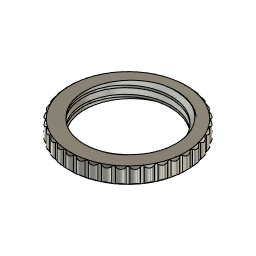
M12x1 knurled thumb nut (Autodesk Fusion 360 design; units mm, degrees)
Autodesk Fusion 360 part; units mm, degrees
sketch "Sketch1" plane through (0, 0, 0) normal (0, 0, 1) x (1, 0, 0)
  circle A0 centre (0, 0) radius 6
  circle A1 centre (0, 0) radius 7.35 construction
  circle A2 centre (0, 0) radius 7.5 construction
  line L0 (0, 0) -> (0, 8.1) construction
  arc A3 (-0.8115, 7.3051) -> (-0.4693, 7.335) centre (-0.6628, 7.5762) ccw
  arc A4 (0, 7.5) -> (-0.4693, 7.335) centre (0, 6.75) ccw
  arc A5 (-0.8115, 7.3051) -> (-1.3024, 7.3861) centre (-1.1721, 6.6475) ccw
  arc A6 (-2.0677, 7.0532) -> (-2.5652, 7.0477) centre (-2.3086, 6.3429) ccw
  arc A7 (-2.0677, 7.0532) -> (-1.7359, 7.1421) centre (-1.9684, 7.346) ccw
  arc A8 (-1.3024, 7.3861) -> (-1.7359, 7.1421) centre (-1.1721, 6.6475) ccw
  arc A9 (-3.261, 6.587) -> (-3.75, 6.4952) centre (-3.375, 5.8457) ccw
  arc A10 (-3.261, 6.587) -> (-2.9497, 6.7321) centre (-3.2141, 6.8926) ccw
  arc A11 (-2.5652, 7.0477) -> (-2.9497, 6.7321) centre (-2.3086, 6.3429) ccw
  arc A12 (-4.3553, 5.9206) -> (-4.8209, 5.7453) centre (-4.3388, 5.1708) ccw
  arc A13 (-4.3553, 5.9206) -> (-4.074, 6.1176) centre (-4.3621, 6.2298) ccw
  arc A14 (-3.75, 6.4952) -> (-4.074, 6.1176) centre (-3.375, 5.8457) ccw
  arc A15 (-5.3173, 5.0744) -> (-5.7453, 4.8209) centre (-5.1708, 4.3388) ccw
  arc A16 (-5.3173, 5.0744) -> (-5.0744, 5.3173) centre (-5.3776, 5.3776) ccw
  arc A17 (-4.8209, 5.7453) -> (-5.0744, 5.3173) centre (-4.3388, 5.1708) ccw
  arc A18 (-6.1176, 4.074) -> (-6.4952, 3.75) centre (-5.8457, 3.375) ccw
  arc A19 (-6.1176, 4.074) -> (-5.9206, 4.3553) centre (-6.2298, 4.3621) ccw
  arc A20 (-5.7453, 4.8209) -> (-5.9206, 4.3553) centre (-5.1708, 4.3388) ccw
  arc A21 (-6.7321, 2.9497) -> (-7.0477, 2.5652) centre (-6.3429, 2.3086) ccw
  arc A22 (-6.7321, 2.9497) -> (-6.587, 3.261) centre (-6.8926, 3.2141) ccw
  arc A23 (-6.4952, 3.75) -> (-6.587, 3.261) centre (-5.8457, 3.375) ccw
  arc A24 (-7.1421, 1.7359) -> (-7.3861, 1.3024) centre (-6.6475, 1.1721) ccw
  arc A25 (-7.1421, 1.7359) -> (-7.0532, 2.0677) centre (-7.346, 1.9684) ccw
  arc A26 (-7.0477, 2.5652) -> (-7.0532, 2.0677) centre (-6.3429, 2.3086) ccw
  arc A27 (-7.335, 0.4693) -> (-7.5, 0) centre (-6.75, 0) ccw
  arc A28 (-7.335, 0.4693) -> (-7.3051, 0.8115) centre (-7.5762, 0.6628) ccw
  arc A29 (-7.3861, 1.3024) -> (-7.3051, 0.8115) centre (-6.6475, 1.1721) ccw
  arc A30 (-7.3051, -0.8115) -> (-7.3861, -1.3024) centre (-6.6475, -1.1721) ccw
  arc A31 (-7.3051, -0.8115) -> (-7.335, -0.4693) centre (-7.5762, -0.6628) ccw
  arc A32 (-7.5, 0) -> (-7.335, -0.4693) centre (-6.75, 0) ccw
  arc A33 (-7.0532, -2.0677) -> (-7.0477, -2.5652) centre (-6.3429, -2.3086) ccw
  arc A34 (-7.0532, -2.0677) -> (-7.1421, -1.7359) centre (-7.346, -1.9684) ccw
  arc A35 (-7.3861, -1.3024) -> (-7.1421, -1.7359) centre (-6.6475, -1.1721) ccw
  arc A36 (-6.587, -3.261) -> (-6.4952, -3.75) centre (-5.8457, -3.375) ccw
  arc A37 (-6.587, -3.261) -> (-6.7321, -2.9497) centre (-6.8926, -3.2141) ccw
  arc A38 (-7.0477, -2.5652) -> (-6.7321, -2.9497) centre (-6.3429, -2.3086) ccw
  arc A39 (-5.9206, -4.3553) -> (-5.7453, -4.8209) centre (-5.1708, -4.3388) ccw
  arc A40 (-5.9206, -4.3553) -> (-6.1176, -4.074) centre (-6.2298, -4.3621) ccw
  arc A41 (-6.4952, -3.75) -> (-6.1176, -4.074) centre (-5.8457, -3.375) ccw
  arc A42 (-5.0744, -5.3173) -> (-4.8209, -5.7453) centre (-4.3388, -5.1708) ccw
  arc A43 (-5.0744, -5.3173) -> (-5.3173, -5.0744) centre (-5.3776, -5.3776) ccw
  arc A44 (-5.7453, -4.8209) -> (-5.3173, -5.0744) centre (-5.1708, -4.3388) ccw
  arc A45 (-4.074, -6.1176) -> (-3.75, -6.4952) centre (-3.375, -5.8457) ccw
  arc A46 (-4.074, -6.1176) -> (-4.3553, -5.9206) centre (-4.3621, -6.2298) ccw
  arc A47 (-4.8209, -5.7453) -> (-4.3553, -5.9206) centre (-4.3388, -5.1708) ccw
  arc A48 (-2.9497, -6.7321) -> (-2.5652, -7.0477) centre (-2.3086, -6.3429) ccw
  arc A49 (-2.9497, -6.7321) -> (-3.261, -6.587) centre (-3.2141, -6.8926) ccw
  arc A50 (-3.75, -6.4952) -> (-3.261, -6.587) centre (-3.375, -5.8457) ccw
  arc A51 (-1.7359, -7.1421) -> (-1.3024, -7.3861) centre (-1.1721, -6.6475) ccw
  arc A52 (-1.7359, -7.1421) -> (-2.0677, -7.0532) centre (-1.9684, -7.346) ccw
  arc A53 (-2.5652, -7.0477) -> (-2.0677, -7.0532) centre (-2.3086, -6.3429) ccw
  arc A54 (-0.4693, -7.335) -> (0, -7.5) centre (0, -6.75) ccw
  arc A55 (-0.4693, -7.335) -> (-0.8115, -7.3051) centre (-0.6628, -7.5762) ccw
  arc A56 (-1.3024, -7.3861) -> (-0.8115, -7.3051) centre (-1.1721, -6.6475) ccw
  arc A57 (0.8115, -7.3051) -> (1.3024, -7.3861) centre (1.1721, -6.6475) ccw
  arc A58 (0.8115, -7.3051) -> (0.4693, -7.335) centre (0.6628, -7.5762) ccw
  arc A59 (0, -7.5) -> (0.4693, -7.335) centre (0, -6.75) ccw
  arc A60 (2.0677, -7.0532) -> (2.5652, -7.0477) centre (2.3086, -6.3429) ccw
  arc A61 (2.0677, -7.0532) -> (1.7359, -7.1421) centre (1.9684, -7.346) ccw
  arc A62 (1.3024, -7.3861) -> (1.7359, -7.1421) centre (1.1721, -6.6475) ccw
  arc A63 (3.261, -6.587) -> (3.75, -6.4952) centre (3.375, -5.8457) ccw
  arc A64 (3.261, -6.587) -> (2.9497, -6.7321) centre (3.2141, -6.8926) ccw
  arc A65 (2.5652, -7.0477) -> (2.9497, -6.7321) centre (2.3086, -6.3429) ccw
  arc A66 (4.3553, -5.9206) -> (4.8209, -5.7453) centre (4.3388, -5.1708) ccw
  arc A67 (4.3553, -5.9206) -> (4.074, -6.1176) centre (4.3621, -6.2298) ccw
  arc A68 (3.75, -6.4952) -> (4.074, -6.1176) centre (3.375, -5.8457) ccw
  arc A69 (5.3173, -5.0744) -> (5.7453, -4.8209) centre (5.1708, -4.3388) ccw
  arc A70 (5.3173, -5.0744) -> (5.0744, -5.3173) centre (5.3776, -5.3776) ccw
  arc A71 (4.8209, -5.7453) -> (5.0744, -5.3173) centre (4.3388, -5.1708) ccw
  arc A72 (6.1176, -4.074) -> (6.4952, -3.75) centre (5.8457, -3.375) ccw
  arc A73 (6.1176, -4.074) -> (5.9206, -4.3553) centre (6.2298, -4.3621) ccw
  arc A74 (5.7453, -4.8209) -> (5.9206, -4.3553) centre (5.1708, -4.3388) ccw
  arc A75 (6.7321, -2.9497) -> (7.0477, -2.5652) centre (6.3429, -2.3086) ccw
  arc A76 (6.7321, -2.9497) -> (6.587, -3.261) centre (6.8926, -3.2141) ccw
  arc A77 (6.4952, -3.75) -> (6.587, -3.261) centre (5.8457, -3.375) ccw
  arc A78 (7.1421, -1.7359) -> (7.3861, -1.3024) centre (6.6475, -1.1721) ccw
  arc A79 (7.1421, -1.7359) -> (7.0532, -2.0677) centre (7.346, -1.9684) ccw
  arc A80 (7.0477, -2.5652) -> (7.0532, -2.0677) centre (6.3429, -2.3086) ccw
  arc A81 (7.335, -0.4693) -> (7.5, 0) centre (6.75, 0) ccw
  arc A82 (7.335, -0.4693) -> (7.3051, -0.8115) centre (7.5762, -0.6628) ccw
  arc A83 (7.3861, -1.3024) -> (7.3051, -0.8115) centre (6.6475, -1.1721) ccw
  arc A84 (7.3051, 0.8115) -> (7.3861, 1.3024) centre (6.6475, 1.1721) ccw
  arc A85 (7.3051, 0.8115) -> (7.335, 0.4693) centre (7.5762, 0.6628) ccw
  arc A86 (7.5, 0) -> (7.335, 0.4693) centre (6.75, 0) ccw
  arc A87 (7.0532, 2.0677) -> (7.0477, 2.5652) centre (6.3429, 2.3086) ccw
  arc A88 (7.0532, 2.0677) -> (7.1421, 1.7359) centre (7.346, 1.9684) ccw
  arc A89 (7.3861, 1.3024) -> (7.1421, 1.7359) centre (6.6475, 1.1721) ccw
  arc A90 (6.587, 3.261) -> (6.4952, 3.75) centre (5.8457, 3.375) ccw
  arc A91 (6.587, 3.261) -> (6.7321, 2.9497) centre (6.8926, 3.2141) ccw
  arc A92 (7.0477, 2.5652) -> (6.7321, 2.9497) centre (6.3429, 2.3086) ccw
  arc A93 (5.9206, 4.3553) -> (5.7453, 4.8209) centre (5.1708, 4.3388) ccw
  arc A94 (5.9206, 4.3553) -> (6.1176, 4.074) centre (6.2298, 4.3621) ccw
  arc A95 (6.4952, 3.75) -> (6.1176, 4.074) centre (5.8457, 3.375) ccw
  arc A96 (5.0744, 5.3173) -> (4.8209, 5.7453) centre (4.3388, 5.1708) ccw
  arc A97 (5.0744, 5.3173) -> (5.3173, 5.0744) centre (5.3776, 5.3776) ccw
  arc A98 (5.7453, 4.8209) -> (5.3173, 5.0744) centre (5.1708, 4.3388) ccw
  arc A99 (4.074, 6.1176) -> (3.75, 6.4952) centre (3.375, 5.8457) ccw
  arc A100 (4.074, 6.1176) -> (4.3553, 5.9206) centre (4.3621, 6.2298) ccw
  arc A101 (4.8209, 5.7453) -> (4.3553, 5.9206) centre (4.3388, 5.1708) ccw
  arc A102 (2.9497, 6.7321) -> (2.5652, 7.0477) centre (2.3086, 6.3429) ccw
  arc A103 (2.9497, 6.7321) -> (3.261, 6.587) centre (3.2141, 6.8926) ccw
  arc A104 (3.75, 6.4952) -> (3.261, 6.587) centre (3.375, 5.8457) ccw
  arc A105 (1.7359, 7.1421) -> (1.3024, 7.3861) centre (1.1721, 6.6475) ccw
  arc A106 (1.7359, 7.1421) -> (2.0677, 7.0532) centre (1.9684, 7.346) ccw
  arc A107 (2.5652, 7.0477) -> (2.0677, 7.0532) centre (2.3086, 6.3429) ccw
  arc A108 (0.4693, 7.335) -> (0, 7.5) centre (0, 6.75) ccw
  arc A109 (0.4693, 7.335) -> (0.8115, 7.3051) centre (0.6628, 7.5762) ccw
  arc A110 (1.3024, 7.3861) -> (0.8115, 7.3051) centre (1.1721, 6.6475) ccw
  dimension "d13" = 12
  dimension "d14" = 14.7
  dimension "d15" = 15
  dimension "d20" = 360
  constraint coincident A0.centre A1.centre
  constraint concentric A0 A1
  constraint vertical L0
  constraint coincident A1 A3.start
  constraint coincident A1 A3.end
  constraint coincident A2 A4.start
  constraint coincident A2 A5.end
  measures "d13" diameter of A0
  measures "d14" diameter of A1
  measures "d15" diameter of A2
extrude "Extrude1" add sketch "Sketch1" along normal blind 2
sketch "Sketch2" plane through (0, 0, 0) normal (0, 1, 0) x (1, 0, 0)
  line L0 (0, 0) -> (0, -2.9) construction
  line L1 (7.335, -2) -> (7.267, -2)
  line L2 (7.335, -2) -> (7.5, -2)
  line L3 (7.267, -2) -> (7.5, -1.767)
  line L4 (7.267, -2) -> (7.6617, -2) construction
  line L5 (7.5, -2) -> (7.5, -1.767)
  line L6 (0.8115, 0) -> (0.8115, -2) construction
  line L7 (0.8115, -1) -> (9, -1) construction
  line L8 (7.335, 0) -> (7.267, 0)
  line L9 (7.267, 0) -> (7.5, -0.233)
  line L10 (7.267, 0) -> (7.6617, 0) construction
  line L11 (7.5, 0) -> (7.5, -0.233)
  line L12 (7.335, 0) -> (7.5, 0)
  dimension "d21" = 45
  constraint coincident L0.start origin
  constraint vertical L0
  constraint horizontal L4
  constraint coincident L1.end L3.start
  constraint coincident L2.end L5.start
  constraint perpendicular L2 L5
  constraint midpoint L6 L7.start
  constraint perpendicular L6 L7
  constraint symmetric L1.start L7 L8.start
  constraint symmetric L1.end L7 L8.end
  constraint symmetric L2.end L7 L11.start
  constraint symmetric L4.end L7 L10.end
  constraint symmetric L3.end L7 L9.end
  measures "d21" angle of L3 L4
revolve "Revolve1" cut sketch "Sketch2" angle 360 about axis through (0, 0, 0) along (0, 0, 1)
thread "Thread2" "ISO Metric profile 12.0 M12x1 6H" major diameter 12.152 minor diameter 11.035 pitch 1 angle 60 modelled right hand crest width 0.2719 on face at (5.9925, -0.2991, 1.3333) crest through (5.5175, 0, 0.25)
